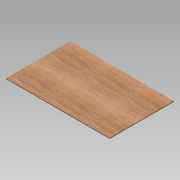
# Autodesk Inventor part: cart_woodpanel-back
Saved by Autodesk Inventor 2015 (Build 190159000, 159)
## iProperties
Created: 2015-05-21
Part Number: cart_woodpanel-back
Material: Wood (Birch)
Document SubType Name: Modeling
Designer: Joe Sheldon
Density: 0.55 g/cm^3
Appearance: Birch - Natural Polished
Author: Joe Sheldon
Autodesk Inventor part; units mm, degrees
ref_plane "YZ Plane" through (0, 0, 0) normal (1, 0, 0) x (0, 1, 0)
ref_plane "XZ Plane" through (0, 0, 0) normal (0, 1, 0) x (-1, 0, 0)
ref_plane "XY Plane" through (0, 0, 0) normal (0, 0, 1) x (1, 0, 0)
sketch "Sketch1" plane through (0, 0, 0) normal (0, 1, 0) x (-1, 0, 0)
  line L0 (0, 0) -> (685.8, 0)
  line L1 (685.8, 0) -> (685.8, -304.8)
  line L2 (685.8, -304.8) -> (0, -304.8)
  line L3 (0, -304.8) -> (0, 0)
  line L4 (685.8, 0) -> (0, 0)
  line L5 (0, 0) -> (0, 120.65)
  line L6 (0, 120.65) -> (685.8, 120.65)
  line L7 (685.8, 120.65) -> (685.8, 0)
  dimension "d0" = 685.8
  dimension "d1" = 304.8
  dimension "d4" = 120.65
  constraints: 16 end point, 4 parallel, 2 horizontal, 2 perpendicular
  measures "d0" distance of L1.end L2.end
  measures "d1" distance of L0.end L1.end
  measures "d4" distance of L4.end L5.end
extrude "Extrusion1" add sketch "Sketch1" along normal blind 5.08 contours L0 L1 L2 L3
sketch "Sketch2" plane through (-685.8, 0, 0) normal (0, 0, 1) x (1, 0, 0)
  line L0 (685.8, 0) -> (0, 0) projected
  line L1 (685.8, 0) -> (685.8, 5.08) projected
  line L2 (0, 5.08) -> (685.8, 5.08) projected
  line L3 (0, 0) -> (0, 5.08) projected
extrude "Extrusion2" add sketch "Sketch2" along normal blind 120.65
sketch "Sketch3" plane through (0, 5.08, 0) normal (0, 1, 0) x (1, 0, 0)
  point P0 (0, 0)
body "Solid1"
